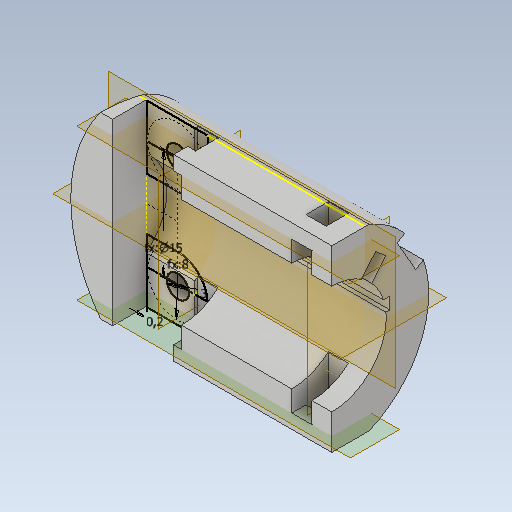
# Autodesk Inventor part: Gimbal_GripHalf_Bottom
Saved by Autodesk Inventor 2021.4 (Build 254397000, 397)
## iProperties
Created: 2022-04-22
Part Number: Gimbal_GripHalf_Bottom
Material: Generisch
Document SubType Name: Modeling
Designer: ALEX
Density: 1 g/cm^3
Appearance: Vorgabe
HollowShaft_Di: 14,600 mm
Hollow_Shaft_Do: 26,000 mm
Flat_Length: 10,000 mm
Author: ALEX
Autodesk Inventor part; units mm, degrees
ref_plane "YZ Plane" through (0, 0, 0) normal (1, 0, 0) x (0, 1, 0)
ref_plane "XY Plane" through (0, 0, 0) normal (0, 0, 1) x (1, 0, 0)
sketch "Skizze1" plane through (0, 0, 0) normal (0, 0, 1) x (1, 0, 0)
  line L0 (0, 0) -> (35, 0) construction
  line L1 (4.8013, 13) -> (35, 13)
  line L2 (35, 13) -> (35, 7.3)
  line L3 (35, 7.3) -> (5.6013, 7.3)
  line L4 (5.6013, 7.3) -> (5.6013, 0)
  arc A0 (4.8013, 13) -> (0, 0) centre (20, 0) ccw
  line L5 (4.8013, 13) -> (4.8013, 0) construction
  line L6 (5.6013, 0) -> (0, 0)
  dimension "HollowShaft_Di" = 14.6
  dimension "Hollow_Shaft_Do" = 26
  dimension "d8" = 20
  dimension "d9" = 0.8
  dimension "GripPart_L" = 35
  constraints: 14 end point, 3 horizontal, 3 perpendicular, 3 point on line, 2 point on circle, 1 centre point, 1 collinear, 1 line through centre
  measures "HollowShaft_Di" diameter of L3 L0
  measures "Hollow_Shaft_Do" diameter of L1 L0
  measures "d8" radius of A0
  measures "d9" distance between parallel lines of L5 L4
  measures "GripPart_L" distance from line of L0.start L2
revolve "Umdrehung1" add sketch "Skizze1" angle 360 about axis through (0, 0, 0) along (1, 0, 0)
sketch "Skizze2" plane through (35, 0, 0) normal (-1, 0, 0) x (0, 0, 1)
  circle A0 centre (0, 0) radius 13 projected
  circle A1 centre (0, 0) radius 13 projected
  line L0 (5, 12) -> (-5, 12)
  line L1 (0, 0) -> (13, 0) construction
  line L2 (5, -12) -> (-5, -12)
  point P0 (0, 0)
  point P1 (5, -12)
  point P2 (-5, -12)
  point P3 (-5, 12)
  point P4 (5, 12)
  dimension "d5" = 10
  constraints: 6 end point, 3 point on circle, 2 horizontal, 2 symmetric about line
  measures "d5" distance of L0.start L0.end
extrude "Flat_extrusion" cut sketch "Skizze2" along normal through all contours L0 A0 | A0 L2
split "Trennen1" plane through (0, 0, 0) removes the side toward (0, 0, 1)
ref_plane "Arbeitsebene2" through (12.25, 0, 0) normal (1, 0, 0) x (0, 0, -1)
ref_plane "Arbeitsebene1" through (32.25, 0, 0) normal (1, 0, 0) x (0, 0, -1)
sketch "Skizze3" plane through (4.8013, 12, -5) normal (0, 1, 0) x (1, 0, 0)
  line L0 (27.4487, 13.2) -> (27.4487, -23.2) construction
  line L1 (7.4487, 13.2) -> (7.4487, -23.2) construction
  line L2 (27.4487, -3) -> (24.9487, -3)
  line L3 (24.9487, -3) -> (24.9487, -0.2)
  line L4 (24.9487, -0.2) -> (27.4487, -0.2)
  line L5 (27.4487, -0.2) -> (27.4487, -3)
  line L6 (-0.8013, -5) -> (30.1987, -5) construction
  line L7 (30.1987, -5) -> (0.8, -5) construction
  line L8 (7.4487, -5) -> (27.4487, -5) construction
  line L9 (17.4487, -5) -> (17.4487, 0) construction
  line L10 (0, 0) -> (30.1987, 0) construction
  line L11 (7.4487, -3) -> (9.9487, -3)
  line L12 (9.9487, -3) -> (9.9487, -0.2)
  line L13 (9.9487, -0.2) -> (7.4487, -0.2)
  line L14 (7.4487, -0.2) -> (7.4487, -3)
  point P0 (-4.8013, -5)
  dimension "d13" = 2.5
  dimension "d14" = 2.8
  dimension "d15" = 2
  constraints: 20 end point, 4 point on line, 4 symmetric about line, 3 midpoint, 2 parallel, 1 horizontal, 1 perpendicular, 1 vertical
  measures "d13" distance of L3.end L4.end
  measures "d14" distance of L2.end L3.end
  measures "d15" distance from line of L6 L2.start
extrude "Extrusion2" cut sketch "Skizze3" against normal through all
ref_plane "Arbeitsebene3" through (4.8013, 10.1, -5) normal (0, 1, 0) x (1, 0, 0)
ref_plane "Arbeitsebene4" through (4.8013, -10.1, -5) normal (0, -1, 0) x (1, 0, 0)
sketch "Skizze4" plane through (4.8013, 10.1, -5) normal (0, 1, 0) x (1, 0, 0)
  line L0 (9.9487, -3) -> (7.4487, -3) projected
  line L1 (-0.8013, -5) -> (30.1987, -5) construction
  line L2 (7.4487, -3) -> (9.9487, -3)
  line L3 (9.9487, -3) -> (9.9487, -5)
  line L4 (9.9487, -5) -> (7.4487, -5)
  line L5 (7.4487, -5) -> (7.4487, -3)
  line L6 (24.9487, -3) -> (24.9487, -0.2) projected
  line L7 (24.9487, -3) -> (27.4487, -3)
  line L8 (27.4487, -3) -> (27.4487, -5)
  line L9 (27.4487, -5) -> (24.9487, -5)
  line L10 (24.9487, -5) -> (24.9487, -3)
  point P0 (-4.8013, -5)
  point P1 (24.9487, 0)
  constraints: 16 end point, 4 parallel, 4 point on line, 2 horizontal, 2 perpendicular
extrude "Extrusion3" cut sketch "Skizze4" against normal up to surface (20.2 mm away)
thicken "SnapAufmass1" operation add thickness 0.1 both sides no extend neighbours yes toward (0, 0, -1) faces at (13.0833, 7.6667, -4.8) (12.25, 9.5269, -3.3868) (14.75, 9.5269, -3.3868) (13.0833, 11.3667, -2)
thicken "SnapAufmass2" operation add thickness 0.1 both sides no extend neighbours yes toward (0, 0, -1) faces at (31.4167, 7.6667, -4.8) (32.25, 9.5269, -3.3868) (29.75, 9.5269, -3.3868) (30.5833, 11.3667, -2)
thicken "SnapAufmass3" operation add thickness 0.1 both sides no extend neighbours yes toward (1, 0, 0) faces at (32.25, -9.5269, -3.3868) (30.5833, -7.6667, -4.8) (29.75, -9.5269, -3.3868) (30.5833, -10.7333, -2)
thicken "SnapAufmass4" operation add thickness 0.1 both sides no extend neighbours yes toward (-1, 0, 0) faces at (12.25, -9.5269, -3.3868) (13.9167, -7.6667, -4.8) (14.75, -9.5269, -3.3868) (13.0833, -10.7333, -2)
ref_plane "Work Plane5" through (4, 12, -4.5) normal (0, 0, 1) x (1, 0, 0)
sketch "LeverFixation" plane through (4, 12, -4.5) normal (0, 0, 1) x (1, 0, 0)
  circle A0 centre (5.8013, -19.5) radius 4 construction
  line L0 (1.6013, -4.7) -> (1.6013, -19.3) construction
  line L1 (31, -24) -> (0.8013, -24) construction
  line L2 (1.6013, -12) -> (5.8013, -12) construction
  circle A1 centre (5.8013, -19.5) radius 1.5
  circle A2 centre (5.8013, -19.5) radius 4 construction
  line L3 (5.8013, -15.5) -> (1.6013, -15.5)
  arc A3 (9.7963, -19.3) -> (5.8013, -15.5) centre (5.8013, -19.5) ccw
  line L4 (1.6013, -19.3) -> (1.6013, -4.7) construction
  circle A4 centre (5.8013, -4.5) radius 4 construction
  circle A5 centre (5.8013, -4.5) radius 1.5
  circle A6 centre (5.8013, -4.5) radius 4 construction
  line L5 (5.8013, -8.5) -> (1.6013, -8.5)
  arc A7 (5.8013, -8.5) -> (9.7963, -4.7) centre (5.8013, -4.5) ccw
  line L6 (5.8013, -19.5) -> (5.8013, -4.5) construction
  line L7 (1.6013, -19.3) -> (31, -19.3) construction
  line L8 (1.6013, -15.5) -> (1.6013, -19.3)
  line L9 (1.6013, -19.3) -> (9.7963, -19.3)
  line L10 (9.7963, -4.7) -> (1.6013, -4.7)
  line L11 (1.6013, -8.5) -> (1.6013, -4.7)
  line L12 (9.7963, -19.3) -> (1.6013, -19.3)
  line L13 (1.6013, -19.3) -> (1.6013, -24)
  line L14 (1.6013, -24) -> (9.7963, -24)
  line L15 (9.7963, -24) -> (9.7963, -19.3)
  line L16 (0.8013, 0) -> (31, 0) projected
  line L17 (1.6013, -4.7) -> (9.7963, -4.7)
  line L18 (9.7963, -4.7) -> (9.7963, 0)
  line L19 (9.7963, 0) -> (1.6013, 0)
  line L20 (1.6013, 0) -> (1.6013, -4.7)
  point P0 (-4, -12)
  point P1 (8.15, -19.3)
  point P2 (7.7946, -4.7)
  point P3 (7.7946, -19.3)
  point P4 (4.3147, -19.3)
  point P5 (7.2879, -19.3)
  point P6 (1.6013, 0)
  point P7 (7.2879, -4.7)
  point P8 (4.3147, -4.7)
  dimension "d31" = 8
  dimension "d32" = 0.2
  dimension "d35" = 15
  dimension "d36" = 3
  constraints: 33 end point, 8 horizontal, 7 symmetric about line, 6 centre point, 5 point on line, 4 coincident, 4 parallel, 4 point on circle, 3 perpendicular, 2 midpoint, 2 vertical alignment, 1 collinear, 1 tangent, 1 vertical, 9 other
  measures "d31" diameter of A0
  measures "d32" distance edge to line of A0 L0
  measures "d35" diameter of A0.centre L2
  measures "d36" diameter of A1
extrude "Lever_Fixation" [suppressed]
extrude "LeverExit" cut sketch "LeverFixation" along normal through all
extrude "Extrusion12" cut sketch "LeverFixation" against normal blind 4 contours A1 L9 | L9 A1 | A5 L10 | L10 A5
sketch "Sketch8" plane through (35, 0, 0) normal (1, 0, 0) x (0, 0, -1)
  line L0 (7.7, 0.75) -> (-8, 0.75) construction
  line L1 (-8, 0.75) -> (-8, 2.15) construction
  line L2 (-8, 2.15) -> (7.7, 2.15) construction
  line L3 (7.7, 2.15) -> (7.7, 0.75) construction
  line L4 (0, 0.75) -> (0, 2.15) construction
  line L5 (-8.1, 0.65) -> (7.8, 0.65)
  line L6 (7.8, 0.65) -> (7.8, 2.25)
  line L7 (7.8, 2.25) -> (-8.1, 2.25)
  line L8 (-8.1, 2.25) -> (-8.1, 0.65)
  point P0 (0, 0)
  dimension "d41" = 1.4
  dimension "d42" = 15.7
  dimension "d43" = 7.7
  dimension "d44" = 0.75
  dimension "d45" = 0.1
  constraints: 18 end point, 4 parallel, 3 perpendicular, 3 point on line, 1 horizontal, 3 other
  measures "d41" distance between parallel lines of L0 L2
  measures "d42" distance between parallel lines of L3 L1
  measures "d43" distance between parallel lines of L3 L4
  measures "d44" distance from line of point (0, 0) L0
  measures "d45" distance between parallel lines of L7 L2
extrude "IMUTrack" cut sketch "Sketch8" against normal blind 20.8
sketch "Sketch9" plane through (35, 0, 0) normal (1, 0, 0) x (0, 0, -1)
  circle A0 centre (0, 0) radius 7.3 construction
  line L0 (-4.6923, -5.5921) -> (4.6923, -5.5921) construction
  line L1 (4.6923, -5.5921) -> (4.6923, 5.5921) construction
  line L2 (4.6923, 5.5921) -> (-4.6923, 5.5921) construction
  line L3 (-4.6923, 5.5921) -> (-4.6923, -5.5921) construction
  line L4 (-4.6923, -5.5921) -> (4.6923, 5.5921) construction
  line L5 (4.6923, -5.5921) -> (-4.6923, 5.5921) construction
  line L6 (0, 0) -> (0, 7.3) construction
  line L7 (3.5177, 2.7921) -> (7.2459, 7.2351) construction
  line L8 (7.2459, 7.2351) -> (5.867, 8.3922) construction
  line L9 (5.867, 8.3922) -> (2.1388, 3.9491) construction
  line L10 (2.1388, 3.9491) -> (3.5177, 2.7921) construction
  line L11 (3.5177, 2.7921) -> (5.867, 8.3922) construction
  line L12 (7.2459, 7.2351) -> (2.1388, 3.9491) construction
  arc A1 (5.346, 4.971) -> (3.9671, 6.128) centre (0, 0) ccw
  line L13 (7.2459, 7.2351) -> (5.867, 8.3922)
  line L14 (7.2459, 7.2351) -> (5.346, 4.971)
  line L15 (5.867, 8.3922) -> (3.9671, 6.128)
  point P0 (0, 0)
  point P1 (4.6923, 5.5921)
  dimension "d48" = 14.6
  dimension "d49" = 40
  dimension "d50" = 1.8
  dimension "d51" = 2.9
  constraints: 32 end point, 7 midpoint, 6 point on circle, 4 parallel, 4 perpendicular, 2 centre point, 2 coincident, 2 point on line, 1 concentric, 1 horizontal, 1 vertical
  measures "d48" diameter of A0
  measures "d49" angle of L6 L5
  measures "d50" distance of L7.end L8.end
  measures "d51" distance from line of L8 point (4.692, 5.592)
extrude "FixationSlide_Track" cut sketch "Sketch9" against normal blind 20.8
ref_plane "Work Plane6" through (0, -8.4167, 0) normal (0, 0, -1) x (0, 1, 0)
sketch "Sketch11" plane through (35, 0, 0) normal (1, 0, 0) x (0, 0, -1)
  line L0 (0, 0) -> (11.2583, 6.5) construction
  arc A0 (5, -12) -> (5, 12) centre (0, 0) ccw construction
  line L1 (0, 0) -> (13, 0) construction
  line L2 (11.259, 3.6136) -> (8.759, 7.9437)
  line L3 (11.259, 3.6136) -> (12.2982, 4.2136)
  line L4 (8.759, 7.9437) -> (9.7982, 8.5437)
  line L5 (12.2982, 4.2136) -> (9.7982, 8.5437) construction
  arc A1 (12.2982, 4.2136) -> (9.7982, 8.5437) centre (0, 0) ccw
  point P0 (10.009, 5.7787)
  dimension "d63" = 30
  dimension "d64" = 1.2
  dimension "d65" = 5
  constraints: 12 end point, 7 point on circle, 4 perpendicular, 1 centre point, 1 midpoint, 1 point on line
  measures "d63" angle of L0 L1
  measures "d64" distance between parallel lines of L2 L5
  measures "d65" distance of L2.start L2.end
extrude "Extrusion9" cut sketch "Sketch11" against normal blind 6
sketch "Sketch12" plane through (35, 3.6136, -11.259) normal (0, 0.5, -0.8660254) x (-1, 0, 0)
  line L0 (6, 0) -> (6, 5) projected
  line L1 (0, 0) -> (6, 0) projected
  line L2 (6, 5) -> (4, 5)
  line L3 (4, 5) -> (4, 0)
  line L4 (4, 0) -> (6, 0)
  line L5 (6, 0) -> (6, 5)
  point P0 (35, 2.5)
  dimension "d68" = 2
  constraints: 8 end point, 2 parallel, 1 horizontal, 1 perpendicular, 1 point on line
  measures "d68" distance between parallel lines of L3 L0
extrude "Extrusion10" cut sketch "Sketch12" against normal blind 1.6
chamfer "Chamfer1" distance 1.2 angle 45 1 edges at (29, 6.5, -11.2583)
equation "\"HollowShaft_Di\" = HollowShaft_Di_1"
equation "\"Hollow_Shaft_Do\" = Hollow_Shaft_Do_1"
equation "\"d5\" = Flat_Length"
equation "\"d13\" = HoleWidth"
equation "\"d14\" = HoleHeight"
equation "\"d15\" = SnapHeight"
equation "\"d22\" = Aufmass"
equation "\"d23\" = Aufmass"
equation "\"d24\" = Aufmass"
equation "\"d25\" = Aufmass"
equation "\"d26\" = Aufmass"
equation "\"d27\" = Aufmass"
equation "\"d28\" = Aufmass"
equation "\"d29\" = Aufmass"
equation "\"d31\" = Lever_Do"
equation "\"d35\" = Hole_Dist"
equation "\"d41\" = BoardThickness"
equation "\"d42\" = B_Frame_Y_top + B_Frame_Y_bottom"
equation "\"d43\" = B_Frame_Y_bottom"
equation "\"d44\" = B_Frame_Z"
equation "\"d45\" = IMU_Aufmass"
equation "\"d46\" = BoardLength"
equation "\"d48\" = HollowShaft_Di_1"
equation "\"d49\" = SlideAngle"
equation "\"d52\" = BoardLength"
equation "\"d63\" = HorizontalSnapper_Angle"
equation "\"d64\" = SnapperThickness"
equation "\"d65\" = SnapperWidth"
equation "\"d66\" = HorizontalSnapper_Length"
equation "\"d68\" = SnapWedge_Width"
equation "\"d69\" = WedgeDepth"
equation "\"d71\" = d64"
equation "\"d11\" = SnapStart"
equation "\"d18\" = -SnapThick"
equation "\"d19\" = -SnapThick"
equation "\"Aufmass\" = 0.1"
equation "\"d30\" = -0.5 * GearThickness"
equation "\"Hole_Dist\" = d"
equation "\"B_Frame_Y_top\" = 8"
equation "\"B_Frame_Y_bottom\" = 7.7"
equation "\"B_Frame_Z\" = 0.75"
equation "\"BoardThickness\" = 1.4"
equation "\"IMU_Aufmass\" = 0.1"
equation "\"HollowShaft_Di_1\" = 14.6"
equation "\"Hollow_Shaft_Do_1\" = 26"
equation "\"Flat_Length\" = 10"
equation "\"HoleWidth\" = 2.5"
equation "\"HoleHeight\" = 2.8"
equation "\"SnapHeight\" = 2"
equation "\"Lever_Do\" = 8"
equation "\"BoardLength\" = 20.8"
equation "\"SlideAngle\" = 40deg"
equation "\"HorizontalSnapper_Angle\" = 30deg"
equation "\"SnapperThickness\" = 1.2"
equation "\"SnapperWidth\" = 5"
equation "\"HorizontalSnapper_Length\" = 6"
equation "\"SnapWedge_Width\" = 2"
equation "\"WedgeDepth\" = 1.6"
equation "\"SnapStart\" = -2.75"
equation "\"SnapThick\" = 1.9"
equation "\"GearThickness\" = 9"
equation "\"d\" = 15"
